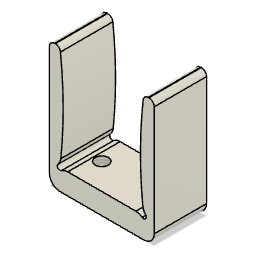
Abrazadera_bateria v6 (Autodesk Fusion 360 design; units mm, degrees)
Autodesk Fusion 360 part; units mm, degrees
note: some values were not read from the file. Set by a fixed rule: which face or edge a step refers to.
sketch "Sketch1" plane through (0, 0, 0) normal (0, 0, 1) x (1, 0, 0)
  line L0 (8, 15) -> (-8, 15)
  line L1 (-8, 15) -> (-8, -15)
  line L2 (-8, -15) -> (8, -15)
  line L3 (8, -15) -> (8, 15)
  line L4 (8, 15) -> (-8, -15) construction
  line L5 (-8, 15) -> (8, -15) construction
  line L6 (-11, 18) -> (-11, -18)
  line L7 (-11, -18) -> (11, -18)
  line L8 (11, -18) -> (11, 18)
  line L9 (11, 18) -> (-11, 18)
  circle A0 centre (-8, -15) radius 0.5
  circle A1 centre (8, -15) radius 0.5
  line L10 (8, 5) -> (11, 5)
  line L11 (0, 0) -> (0, 18) construction
  line L12 (-8, 5) -> (-11, 5)
  line L13 (-11, -5) -> (11, -5) construction
  arc A2 (-8, -15) -> (-8, 5) centre (-88, -5) ccw
  line L14 (7.5, 10) -> (-7.5, 10) construction
  line L15 (-7.5, 10) -> (-7.5, -10) construction
  line L16 (-7.5, -10) -> (7.5, -10) construction
  line L17 (7.5, -10) -> (7.5, 10) construction
  line L18 (7.5, 10) -> (-7.5, -10) construction
  line L19 (-7.5, 10) -> (7.5, -10) construction
  arc A3 (8, 5) -> (8, -15) centre (88, -5) ccw
  dimension "d1" = 16
  dimension "d2" = 30
  dimension "d3" = 3
  dimension "d4" = 1
  dimension "d5" = 5
  dimension "d20" = 5
  dimension "d21" = 80
  dimension "d22" = 15
  dimension "d23" = 20
  constraint horizontal L0
  constraint perpendicular L0 L1
  constraint parallel L0 L2
  constraint parallel L1 L3
  constraint coincident L4 L11.start
  constraint coincident L5 L11.start
  constraint coincident L11.start origin
  constraint coincident L1.end L2.start
  constraint coincident L2.end L3.start
  constraint equal A0 A1
  constraint coincident L3 L10.start
  constraint coincident L8 L10.end
  constraint perpendicular L3 L10
  constraint midpoint L9 L11.end
  constraint symmetric L10.start L11 L12.start
  constraint symmetric L10.end L11 L12.end
  constraint coincident L6 L13.start
  constraint coincident L8 L13.end
  constraint perpendicular L8 L13
  constraint horizontal L14
  constraint perpendicular L14 L15
  constraint parallel L14 L16
  constraint parallel L15 L17
  constraint coincident L18 L11.start
  constraint coincident L19 L11.start
  constraint symmetric L11 L12.start L10.start
  constraint symmetric L11 L1.end L2.end
  constraint symmetric L11 A2 A3
  measures "d1" distance of L1.end L2.end
  measures "d2" distance of L0.start L2.end
  measures "d4" diameter of A0
  measures "d5" distance of L11.start L10
  measures "d20" distance of L11.start L13
  measures "d21" distance of L1 A2.centre
  measures "d22" distance of L15.end L16.end
  measures "d23" distance of L14.end L15.end
extrude "Extrude1" add sketch "Sketch1" along normal mid plane 10 contours L1 L2 L3 L6 L7 L8 A0 A1 L10 L12 | L3 A1 A3 | L1 A0 A2 picked at (7.8179, -3.6642) picked at (-7.8179, -3.6642)
fillet "Fillet1" radius 2 2 edges at (-11, -18, 0) (11, -18, 0)
fillet "Fillet2" radius 2 4 edges at (7.5, -15, 0) (-7.5, -15, 0) (-7.9395, -14.5037, 0) (7.9395, -14.5037, 0)
sketch "Sketch2" plane through (0, -18, 0) normal (0, -1, 0) x (1, 0, 0)
  line L0 (9, -5) -> (9, 5)
  line L1 (9, 5) -> (-9, 5)
  line L2 (-9, 5) -> (-9, -5)
  line L3 (-9, -5) -> (9, -5)
  line L4 (5, 3) -> (-5, 3) construction
  line L5 (-5, 3) -> (-5, -3) construction
  line L6 (-5, -3) -> (5, -3) construction
  line L7 (5, -3) -> (5, 3) construction
  line L8 (5, 3) -> (-5, -3) construction
  line L9 (-5, 3) -> (5, -3) construction
  circle A0 centre (5, 3) radius 1.5 construction
  circle A1 centre (5, -3) radius 1.5 construction
  line L10 (0, 0) -> (0, 3) construction
  circle A2 centre (-5, 3) radius 1.5 construction
  circle A3 centre (-5, -3) radius 1.5 construction
  circle A4 centre (5, 0) radius 1.5
  circle A5 centre (-5, 0) radius 1.5
  dimension "d12" = 3
  dimension "d13" = 3
  dimension "d14" = 6
  dimension "d15" = 10
  dimension "d18" = 3
  dimension "d19" = 3
  constraint horizontal L4
  constraint perpendicular L4 L5
  constraint parallel L4 L6
  constraint parallel L5 L7
  constraint coincident L8 L10.start
  constraint coincident L9 L10.start
  constraint coincident L10.start origin
  constraint coincident L4.start L7.end
  constraint coincident L6.end L7.start
  constraint midpoint L4 L10.end
  constraint symmetric A0 L10 A2
  constraint symmetric A1 L10 A3
  constraint midpoint L7 A4.centre
  constraint midpoint L5 A5.centre
  measures "d12" diameter of A0
  measures "d13" diameter of A1
  measures "d14" distance of L4.start L6.end
  measures "d15" distance of L5.end L6.end
  measures "d18" diameter of A4
  measures "d19" diameter of A5
extrude "Extrude2" cut sketch "Sketch2" against normal blind 4 contours A4 | A5
move_face "OffsetFaces1" offset 1 1 faces at (1.484, -18, -3.7988)
move_face "OffsetFaces2" offset -1 2 faces at (11, -9.6667, 1.6667) (-11, -2.3333, 1.6667)
thread "Thread1" "ISO Metric profile 3.0 M3x0.5 6H" major diameter 3.086 minor diameter 2.529 pitch 0.5 angle 60 resizes the face on face at (-3.5075, -18.3333, -0.1494) on face at (-3.5019, -16, -0.0748) on face at (6.4925, -18.3333, -0.1494) on face at (6.4925, -16, -0.1494)
fillet "Fillet3" radius 1 4 edges at (-8, 5, 0) (-10, 5, 0) (8, 5, 0) (10, 5, 0)
